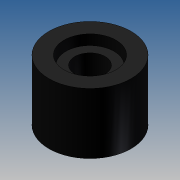
# Autodesk Inventor part: staklence
Saved by Autodesk Inventor 2014 (Build 180170000, 170)
## iProperties
Created: 2011-11-30
Part Number: staklence
Material: Generic
Document SubType Name: Modeling
Designer: slazh bliskovic
Density: 1 g/cm^3
Mass: 0.724085 g
Surface Area: 9.78933 cm^2
Volume: 0.724085 cm^3
Appearance: Glossy - Black
Author: slazh bliskovic
Autodesk Inventor part; units mm, degrees
ref_plane "YZ Plane" through (0, 0, 0) normal (1, 0, 0) x (0, 1, 0)
ref_plane "XZ Plane" through (0, 0, 0) normal (0, 1, 0) x (-1, 0, 0)
ref_plane "XY Plane" through (0, 0, 0) normal (0, 0, 1) x (1, 0, 0)
sketch "Sketch1" plane through (0, 0, 0) normal (0, 0, 1) x (1, 0, 0)
  circle A0 centre (0, 0) radius 1.5
  circle A1 centre (0, 0) radius 2.125
  circle A2 centre (0, 0) radius 3.375
  circle A3 centre (0, 0) radius 3.625
  circle A4 centre (0, 0) radius 5.75
  dimension "d0" = 3
  dimension "d1" = 4.25
  dimension "d2" = 6.75
  dimension "d3" = 7.25
  dimension "d4" = 11.5
  constraints: 5 centre point, 5 coincident
  measures "d0" diameter of A0
  measures "d1" diameter of A1
  measures "d2" diameter of A2
  measures "d3" diameter of A3
  measures "d4" diameter of A4
extrude "Extrusion1" add sketch "Sketch1" along normal blind 8.5
sketch "Sketch2" plane through (0, 0, 0) normal (1, 0, 0) x (0, 1, 0)
  line L0 (-1.5, 8.5) -> (1.5, 8.5) construction
  line L1 (-3.4583, 7.2567) -> (-1.856, 7.2567) construction
  line L2 (-1.856, 7.2567) -> (-1.856, 5.2471) construction
  line L3 (-1.856, 5.2471) -> (0, 5.2471) construction
  line L4 (-3.4583, 7.2567) -> (-3.4583, 8.9404)
  line L5 (-3.4583, 8.9404) -> (0, 8.9404)
  line L6 (0, 8.9404) -> (0, 5.2471)
  line L7 (0, 5.2471) -> (-1.856, 5.2471)
  line L8 (-1.856, 5.2471) -> (-1.856, 7.2567)
  line L9 (-1.856, 7.2567) -> (-3.4583, 7.2567)
  point P0 (0, 0)
  constraints: 18 end point, 3 collinear, 3 parallel, 3 perpendicular
revolve "Revolution1" cut sketch "Sketch2" angle 360 about axis through (0, 0, 8.9404) along (0, 0, -1)
fillet "Fillet1" radius 1 1 edges at (-1.5, 0, 5.2471)
body "Solid1"
